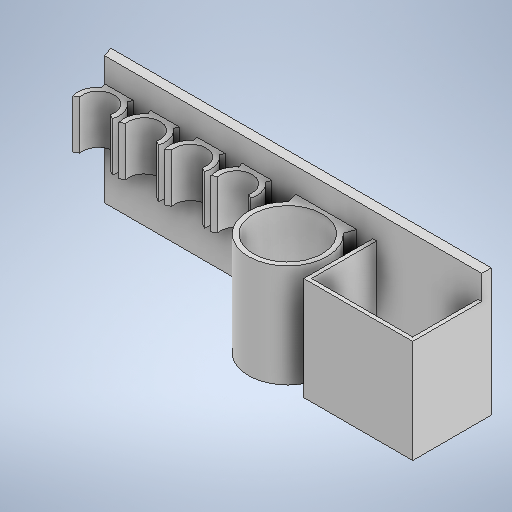
# Autodesk Inventor part: Block-1
Saved by Autodesk Inventor 2025 (Build 290162000, 162)
## iProperties
Created: 2024-07-25
Part Number: Block-1
Material: Generic
Document SubType Name: Modeling
Designer: ethan
Density: 1 g/cm^3
Appearance: Default
Author: ethan
Autodesk Inventor part; units mm, degrees
ref_plane "YZ Plane" through (0, 0, 0) normal (1, 0, 0) x (0, 1, 0)
ref_plane "XZ Plane" through (0, 0, 0) normal (0, 1, 0) x (-1, 0, 0)
ref_plane "XY Plane" through (0, 0, 0) normal (0, 0, 1) x (1, 0, 0)
sketch "Sketch1" plane through (0, 0, 0) normal (0, 1, 0) x (-1, 0, 0)
  arc A0 (-1.6722, -8.0788) -> (-1.6722, 8.0788) centre (0, 0) ccw
  arc A1 (-2.9725, -10.3309) -> (-2.9725, 10.3309) centre (0, 0) ccw
  line L0 (-1.6722, 8.0788) -> (-2.9725, 10.3309)
  line L1 (-1.6722, 8.0788) -> (0.9283, 8.0788) construction
  line L2 (-1.6722, -8.0788) -> (-2.9725, -10.3309)
  line L3 (0, 0) -> (0, -2.9706)
  arc A2 (-1.6722, -32.0788) -> (-1.6722, -15.9212) centre (0, -24) ccw
  arc A3 (-2.9725, -34.3309) -> (-2.9725, -13.6691) centre (0, -24) ccw
  line L4 (-1.6722, -15.9212) -> (-2.9725, -13.6691)
  line L5 (-1.6722, -15.9212) -> (0.9283, -15.9212) construction
  line L6 (-1.6722, -32.0788) -> (-2.9725, -34.3309)
  line L7 (0, -24) -> (0, -26.9706)
  arc A4 (-1.6722, -56.0788) -> (-1.6722, -39.9212) centre (0, -48) ccw
  arc A5 (-2.9725, -58.3309) -> (-2.9725, -37.6691) centre (0, -48) ccw
  line L8 (-1.6722, -39.9212) -> (-2.9725, -37.6691)
  line L9 (-1.6722, -39.9212) -> (0.9283, -39.9212) construction
  line L10 (-1.6722, -56.0788) -> (-2.9725, -58.3309)
  line L11 (0, -48) -> (0, -50.9706)
  arc A6 (-1.6722, -80.0788) -> (-1.6722, -63.9212) centre (0, -72) ccw
  arc A7 (-2.9725, -82.3309) -> (-2.9725, -61.6691) centre (0, -72) ccw
  line L12 (-1.6722, -63.9212) -> (-2.9725, -61.6691)
  line L13 (-1.6722, -63.9212) -> (0.9283, -63.9212) construction
  line L14 (-1.6722, -80.0788) -> (-2.9725, -82.3309)
  line L15 (0, -72) -> (0, -74.9706)
  line L16 (10.75, -134.4179) -> (-23.25, -134.4179)
  line L17 (-23.25, -134.4179) -> (-23.25, -187.2179)
  line L18 (-23.25, -187.2179) -> (10.75, -187.2179)
  line L19 (10.75, -187.2179) -> (10.75, -134.4179)
  line L20 (-25.25, -189.2179) -> (-25.25, -132.4179)
  line L21 (-25.25, -132.4179) -> (10.75, -132.4179)
  line L22 (12.75, -189.2179) -> (-25.25, -189.2179)
  line L23 (10.75, 0) -> (15.75, 0) construction
  line L24 (8.4709, 6.6186) -> (15.75, 9.268) construction
  line L25 (15.75, 9.268) -> (15.75, -189.2179) construction
  line L26 (15.75, -189.2179) -> (12.75, -189.2179) construction
  line L27 (10.75, -132.4179) -> (10.75, -124.0159) construction
  line L28 (10.75, -132.4179) -> (10.75, -124.0159)
  line L29 (10.75, -92.1105) -> (10.75, -79.8019)
  line L30 (8.4709, 6.6186) -> (15.75, 9.268)
  line L31 (15.75, 9.268) -> (15.75, -189.2179)
  line L32 (15.75, -189.2179) -> (12.75, -189.2179)
  line L33 (10.75, -124.0159) -> (10.75, -132.4179) construction
  line L34 (10.75, -134.4179) -> (10.75, -154.7804) construction
  line L35 (8.4709, -6.6186) -> (10.75, -7.4481)
  line L36 (8.4709, -6.6186) -> (10.8963, -6.6186) construction
  line L37 (8.4709, -17.3814) -> (10.75, -16.5519)
  line L38 (8.4709, -30.6186) -> (10.75, -31.4481)
  line L39 (8.4709, -41.3814) -> (10.75, -40.5519)
  line L40 (8.4709, -54.6186) -> (10.75, -55.4481)
  line L41 (8.25, -65.108) -> (10.75, -64.1981)
  line L42 (8.25, -78.892) -> (10.75, -79.8019)
  line L43 (10.75, -16.5519) -> (10.75, -7.4481)
  line L44 (10.75, -7.4481) -> (10.75, -16.5519) construction
  line L45 (10.75, -64.1981) -> (10.75, -55.4481)
  line L46 (10.75, -40.5519) -> (10.75, -31.4481)
  line L47 (10.75, -31.4481) -> (10.75, -40.5519) construction
  line L48 (10.75, -55.4481) -> (10.75, -64.1981) construction
  line L49 (10.75, -79.8019) -> (10.75, -92.1105) construction
  line L50 (8.75, -108.0632) -> (-9.25, -108.0632) construction
  arc A8 (5.4844, -93.8102) -> (5.4844, -122.3162) centre (-9.25, -108.0632) ccw construction
  arc A9 (5.4844, -93.8102) -> (5.4844, -122.3162) centre (-9.25, -108.0632) ccw construction
  circle A10 centre (-9.25, -108.0632) radius 18 construction
  line L51 (5.4844, -93.8102) -> (10.75, -92.1105) construction
  line L52 (10.75, -94.1578) -> (11.111, -94.1578) construction
  line L53 (5.4844, -122.3162) -> (10.75, -124.0159) construction
  line L54 (10.75, -121.9686) -> (11.111, -121.9686) construction
  line L55 (10.75, -92.1105) -> (5.4844, -93.8102)
  line L56 (5.4844, -122.3162) -> (10.75, -124.0159)
  circle A11 centre (-9.25, -108.0632) radius 18
  arc A12 (5.4844, -93.8102) -> (5.4844, -122.3162) centre (-9.25, -108.0632) ccw
  dimension "d1" = 2.5
  dimension "d5" = 24
  dimension "d19" = 20
  dimension "d31" = 2
  dimension "d32" = 34
  dimension "d33" = 52.8
  dimension "d34" = 2
  dimension "d43" = 2.5
  dimension "d44" = 2
  dimension "d45" = 5
  constraints: 114 end point, 31 point on circle, 30 collinear, 12 centre point, 12 tangent, 10 parallel, 9 perpendicular, 9 vertical, 7 coincident, 6 horizontal, 2 equal length, 1 horizontal alignment, 1 point on line, 47 other
  measures "d1" radial gap between concentric circles of A0 A1
  measures "d5" distance of point (0, 0) point (0, -24)
  measures "d19" angle of L35 L36
  measures "d31" distance between parallel lines of L16 L21
  measures "d32" distance of L16.start L16.end
  measures "d33" distance between parallel lines of L18 L16
  measures "d34" distance between parallel lines of L22 L18
  measures "d44" distance between parallel lines of L17 L20
  measures "d45" distance between parallel lines of L25 L19
extrude "Extrusion1" add sketch "Sketch1" along normal blind 25.4
sketch "Sketch6" plane through (0, 25.4, 0) normal (0, 1, 0) x (1, 0, 0)
  line L0 (-15.75, 189.2179) -> (-15.75, -9.268) projected
  line L1 (25.25, 189.2179) -> (-15.75, 189.2179) projected
  line L2 (-15.75, -9.268) -> (-8.4709, -6.6186) projected
  line L3 (-10.75, 134.4179) -> (-10.75, 187.2179) projected
  line L4 (-15.75, 189.2179) -> (-10.75, 189.2179)
  line L5 (-10.75, 189.2179) -> (-10.75, -15.2397)
  line L6 (-10.75, -15.2397) -> (-15.75, -15.2397)
  line L7 (-15.75, -15.2397) -> (-15.75, 189.2179)
  point P0 (0, 0)
  point P1 (-10.75, -7.4481)
  constraints: 8 end point, 2 parallel, 1 horizontal, 1 perpendicular
extrude "Extrusion6" add sketch "Sketch6" along normal blind 12.7 contours L1 L5 L3 L2 L0
sketch "Sketch7" plane through (0, 0, 0) normal (0, -1, 0) x (1, 0, 0)
  line L0 (-10.75, -124.0159) -> (-10.75, -92.1105) construction
  arc A0 (1.6722, -15.9212) -> (1.6722, -32.0788) centre (0, -24) ccw construction
  line L1 (2.9725, -13.6691) -> (1.6722, -15.9212) construction
  arc A1 (2.9725, -13.6691) -> (-8.4709, -17.3814) centre (0, -24) ccw construction
  line L2 (-10.75, -16.5519) -> (-8.4709, -17.3814) construction
  line L3 (-10.75, -7.4481) -> (-10.75, -16.5519) construction
  line L4 (-8.4709, -6.6186) -> (-10.75, -7.4481) construction
  arc A2 (-8.4709, -6.6186) -> (2.9725, -10.3309) centre (0, 0) ccw construction
  line L5 (1.6722, -8.0788) -> (2.9725, -10.3309) construction
  arc A3 (1.6722, 8.0788) -> (1.6722, -8.0788) centre (0, 0) ccw construction
  line L6 (2.9725, 10.3309) -> (1.6722, 8.0788) construction
  arc A4 (2.9725, 10.3309) -> (-8.4709, 6.6186) centre (0, 0) ccw construction
  line L7 (-15.75, 9.268) -> (-8.4709, 6.6186) construction
  line L8 (-15.75, -189.2179) -> (-15.75, 9.268) construction
  line L9 (25.25, -189.2179) -> (-15.75, -189.2179) construction
  line L10 (25.25, -132.4179) -> (25.25, -189.2179) construction
  line L11 (-10.75, -132.4179) -> (25.25, -132.4179) construction
  line L12 (-10.75, -124.0159) -> (-10.75, -132.4179) construction
  line L13 (-5.4844, -122.3162) -> (-10.75, -124.0159) construction
  arc A5 (-5.4844, -122.3162) -> (-5.4844, -93.8102) centre (9.25, -108.0632) ccw construction
  line L14 (-10.75, -92.1105) -> (-5.4844, -93.8102) construction
  line L15 (-10.75, -79.8019) -> (-10.75, -92.1105) construction
  line L16 (-8.25, -78.892) -> (-10.75, -79.8019) construction
  arc A6 (-8.25, -78.892) -> (2.9725, -82.3309) centre (0, -72) ccw construction
  line L17 (1.6722, -80.0788) -> (2.9725, -82.3309) construction
  arc A7 (1.6722, -63.9212) -> (1.6722, -80.0788) centre (0, -72) ccw construction
  line L18 (2.9725, -61.6691) -> (1.6722, -63.9212) construction
  arc A8 (2.9725, -61.6691) -> (-8.25, -65.108) centre (0, -72) ccw construction
  line L19 (-10.75, -64.1981) -> (-8.25, -65.108) construction
  line L20 (-10.75, -55.4481) -> (-10.75, -64.1981) construction
  line L21 (-8.4709, -54.6186) -> (-10.75, -55.4481) construction
  arc A9 (-8.4709, -54.6186) -> (2.9725, -58.3309) centre (0, -48) ccw construction
  line L22 (1.6722, -56.0788) -> (2.9725, -58.3309) construction
  arc A10 (1.6722, -39.9212) -> (1.6722, -56.0788) centre (0, -48) ccw construction
  line L23 (2.9725, -37.6691) -> (1.6722, -39.9212) construction
  arc A11 (2.9725, -37.6691) -> (-8.4709, -41.3814) centre (0, -48) ccw construction
  line L24 (-10.75, -40.5519) -> (-8.4709, -41.3814) construction
  line L25 (-10.75, -31.4481) -> (-10.75, -40.5519) construction
  line L26 (-8.4709, -30.6186) -> (-10.75, -31.4481) construction
  arc A12 (-8.4709, -30.6186) -> (2.9725, -34.3309) centre (0, -24) ccw construction
  line L27 (1.6722, -32.0788) -> (2.9725, -34.3309) construction
  circle A13 centre (9.25, -108.0632) radius 18 construction
  line L28 (-10.75, -134.4179) -> (-10.75, -187.2179) construction
  line L29 (23.25, -134.4179) -> (-10.75, -134.4179) construction
  line L30 (23.25, -187.2179) -> (23.25, -134.4179) construction
  line L31 (-10.75, -187.2179) -> (23.25, -187.2179) construction
  line L32 (-10.75, -189.2179) -> (-15.75, -189.2179)
  line L33 (-15.75, -189.2179) -> (-15.75, 9.268)
  line L34 (-15.75, -189.2179) -> (25.25, -189.2179)
  line L35 (25.25, -189.2179) -> (25.25, -132.4179)
  line L36 (25.25, -132.4179) -> (-10.75, -132.4179)
  line L37 (-15.75, -132.4179) -> (-15.75, -189.2179)
  line L38 (23.25, -134.4179) -> (-10.75, -134.4179)
  line L39 (-10.75, -134.4179) -> (-10.75, -187.2179)
  line L40 (-10.75, -187.2179) -> (23.25, -187.2179)
  line L41 (23.25, -187.2179) -> (23.25, -134.4179)
  circle A14 centre (9.25, -108.0632) radius 18
  arc A15 (-5.4844, -122.3162) -> (-5.4844, -93.8102) centre (9.25, -108.0632) ccw
  line L42 (-10.75, -92.1105) -> (-5.4844, -93.8102)
  line L43 (-10.75, -124.0159) -> (-5.4844, -122.3162)
  line L44 (-15.75, 9.268) -> (-10.75, 7.4481)
  line L45 (-10.75, 7.4481) -> (-10.75, -92.1105)
  line L46 (-10.75, -124.0159) -> (-10.75, -132.4179)
  line L47 (-10.75, -134.4179) -> (-10.75, -187.2179)
  constraints: 32 end point, 7 parallel, 5 point on line, 2 centre point, 2 coincident, 2 concentric, 2 horizontal, 2 perpendicular, 2 point on circle, 1 collinear
extrude "Extrusion7" add sketch "Sketch7" along normal blind 25.4
sketch "Sketch8" plane through (0, -25.4, 0) normal (0, -1, 0) x (1, 0, 0)
  line L0 (25.25, -132.4179) -> (-10.75, -132.4179) projected
  line L1 (-10.75, -132.4179) -> (-10.75, -124.0159) projected
  line L2 (-10.75, -124.0159) -> (-5.4844, -122.3162) projected
  arc A0 (-5.4844, -122.3162) -> (-5.4844, -93.8102) centre (9.25, -108.0632) ccw projected
  line L3 (-5.4844, -93.8102) -> (-10.75, -92.1105) projected
  line L4 (-10.75, -92.1105) -> (-10.75, 7.4481) projected
  line L5 (-10.75, 7.4481) -> (-15.75, 9.268) projected
  line L6 (-15.75, 9.268) -> (-15.75, -189.2179) projected
  line L7 (-15.75, -189.2179) -> (25.25, -189.2179) projected
  line L8 (25.25, -189.2179) -> (25.25, -132.4179) projected
  circle A1 centre (9.25, -108.0632) radius 18 projected
  line L9 (-10.75, -134.4179) -> (23.25, -134.4179) projected
  line L10 (23.25, -134.4179) -> (23.25, -187.2179) projected
  line L11 (23.25, -187.2179) -> (-10.75, -187.2179) projected
  line L12 (-10.75, -187.2179) -> (-10.75, -134.4179) projected
  point P0 (0, 0)
extrude "Extrusion8" add sketch "Sketch8" along normal blind 3 contours L8 L7 L6 L5 L4 L3 A0 L2 L1 L0 | A1 | L9 L10 L11 L12
body "Solid1"
